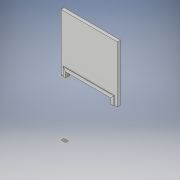
# Autodesk Inventor part: door-frame
Saved by Autodesk Inventor 2018 (Build 220112000, 112)
## iProperties
Created: 2018-11-24
Part Number: door-frame
Material: Generic
Document SubType Name: Modeling
Designer: Gage
Density: 1 g/cm^3
Appearance: Default
Author: Gage
Autodesk Inventor part; units mm, degrees
ref_plane "YZ Plane" through (0, 0, 0) normal (1, 0, 0) x (0, 1, 0)
ref_plane "XZ Plane" through (0, 0, 0) normal (0, 1, 0) x (-1, 0, 0)
sketch "Sketch1" plane through (0, 0, 0) normal (0, 0, 1) x (1, 0, 0)
  line L0 (-12.7, 38.1) -> (12.7, 38.1)
  line L1 (12.7, 38.1) -> (12.7, -38.1)
  line L2 (12.7, -38.1) -> (-12.7, -38.1)
  line L3 (-12.7, -38.1) -> (-12.7, 38.1)
  line L4 (-12.7, 38.1) -> (12.7, -38.1) construction
  line L5 (12.7, 38.1) -> (-12.7, -38.1) construction
  point P0 (0, 0)
  dimension "d0" = 25.4
  dimension "d1" = 76.2
  constraints: 12 end point, 2 midpoint, 2 parallel, 1 horizontal, 1 perpendicular
  measures "d0" distance of L1.end L2.end
  measures "d1" distance of L0.end L1.end
extrude "Extrusion1" add sketch "Sketch1" along normal blind 1.397
sketch "Sketch2" plane through (0, 0, 1.397) normal (0, 0, 1) x (1, 0, 0)
  line L0 (-10.16, -38.1) -> (10.16, -38.1)
  line L1 (10.16, -38.1) -> (10.16, 15.24)
  line L2 (10.16, 15.24) -> (-10.16, 15.24)
  line L3 (-10.16, 15.24) -> (-10.16, -38.1)
  line L4 (-12.7, -38.1) -> (12.7, -38.1) projected
  point P0 (0, 0)
  point P1 (0, -38.1)
  dimension "d4" = 20.32
  dimension "d5" = 53.34
  constraints: 8 end point, 2 midpoint, 2 parallel, 1 horizontal, 1 perpendicular
  measures "d4" distance of L2.end L1.end
  measures "d5" distance of L1.end L0.end
extrude "Extrusion2" cut sketch "Sketch2" against normal through all
sketch "Sketch3" plane through (12.7, -38.1, 0) normal (1, 0, 0) x (0, 0, -1)
  line L0 (0, 76.2) -> (0, 0) projected
  line L1 (0, 76.2) -> (-1.397, 76.2) projected
  line L2 (-1.397, 0) -> (-1.397, 76.2) projected
  line L3 (0, 0) -> (-1.397, 0) projected
  line L4 (-1.397, 0) -> (-1.905, 0)
  line L5 (-1.397, 0) -> (-1.397, 1.27)
  line L6 (-1.397, 53.34) -> (-1.397, 0) projected
  line L7 (-1.651, 1.27) -> (-1.397, 1.27)
  line L8 (-1.651, 1.27) -> (-1.905, 0)
  point P0 (0, 38.1)
  dimension "d8" = 0.508
  dimension "d9" = 1.27
  dimension "d10" = 0.254
  constraints: 8 end point, 2 horizontal, 1 collinear
  measures "d8" distance of L2.start L4.end
  measures "d9" distance of L2.start L5.end
  measures "d10" distance of L7.start L5.end
ref_plane "Work Plane1" through (0, 0, 1.651) normal (0, 0, 1) x (1, 0, 0)
sketch "Sketch6" plane through (0, 0, 1.651) normal (0, 0, 1) x (1, 0, 0)
  line L0 (12.7, -36.83) -> (12.7, -38.1) projected
  line L1 (12.7, -38.1) -> (12.7, 38.1) projected
  line L2 (12.7, -37.465) -> (10.795, -37.465)
  line L3 (10.16, -38.1) -> (12.7, -38.1) projected
  line L4 (10.16, 15.24) -> (10.16, -38.1) projected
  line L5 (10.795, -37.465) -> (10.795, 15.875)
  line L6 (10.795, 15.875) -> (-10.795, 15.875)
  line L7 (-10.795, 15.875) -> (-10.795, -37.465)
  line L8 (-10.795, -37.465) -> (-12.7255, -37.465)
  line L9 (-12.7, -38.1) -> (-10.16, -38.1) projected
  line L10 (-10.16, -38.1) -> (-10.16, 15.24) projected
  line L11 (-10.16, 15.24) -> (10.16, 15.24) projected
  point P0 (0, 0)
  dimension "d12" = 0.635
  dimension "d13" = 0.635
  dimension "d14" = 0.635
  dimension "d15" = 0.635
  dimension "d16" = 0.635
  constraints: 10 end point, 2 horizontal, 2 perpendicular, 1 parallel, 1 point on line
  measures "d12" distance between parallel lines of L3 L2
  measures "d13" distance from line of L4 L2.end
  measures "d14" distance between parallel lines of L9 L8
  measures "d15" distance between parallel lines of L10 L7
  measures "d16" distance between parallel lines of L11 L6
sweep "Sweep1" add profiles "Sketch3" path "Sketch6" path curves L2 L5 L6 L7 L8 contours L4 L8 L7 L2
ref_plane "Work Plane3" through (-12.7, 12.7, 0) normal (0, -1, 0) x (1, 0, 0)
ref_plane "Work Plane2" through (-12.7, -12.7, 0) normal (0, -1, 0) x (1, 0, 0)
split "Split3" plane through (-12.7, -12.7, 0) removes the side toward (0, -1, 0)
split "Split5" plane through (-12.7, 12.7, 0) removes the side toward (0, -1, 0)
body "Solid1"
